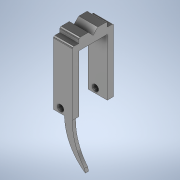
# Autodesk Inventor part: Part2
Saved by Autodesk Inventor 2021 (Build 250183000, 183)
## iProperties
Created: 2020-11-21
Part Number: Part2
Material: Nickel-Copper Alloy 400
Document SubType Name: Modeling
Designer: pedro
Density: 8.83 g/cm^3
Appearance: Cromado - Preto polido
Author: pedro
Autodesk Inventor part; units mm, degrees
ref_plane "YZ Plane" through (0, 0, 0) normal (1, 0, 0) x (0, 1, 0)
ref_plane "XZ Plane" through (0, 0, 0) normal (0, 1, 0) x (-1, 0, 0)
ref_plane "XY Plane" through (0, 0, 0) normal (0, 0, 1) x (1, 0, 0)
sketch "Sketch1" plane through (0, 0, 0) normal (0, 0, 1) x (1, 0, 0)
  line L0 (0, 0) -> (-5, 0)
  line L1 (-5, 0) -> (-5, 20)
  line L2 (-5, 20) -> (0, 20)
  line L3 (0, 20) -> (0, 0)
  arc A0 (0, 0) -> (3.7628, -11.2711) centre (16.9897, -0.5917) ccw
  arc A1 (-2.5, 0) -> (3.7698, -12.1977) centre (12.5, 0) ccw
  line L4 (4.0643, -12.4032) -> (3.7628, -11.2711)
  line L5 (-5, 0) -> (-2.5, 0)
  line L6 (0, 20) -> (0, 0)
  line L7 (3.7698, -12.1977) -> (4.0643, -12.4032)
  circle A2 centre (-3.75, 1.4711) radius 1.0155
  dimension "d0" = 5
  dimension "d1" = 20
  dimension "d2" = 17
  dimension "d3" = 15
  constraints: 16 end point, 5 point on circle, 3 centre point, 2 parallel, 2 perpendicular, 1 collinear, 1 horizontal, 1 midpoint
  measures "d0" distance of L1.end L2.end
  measures "d1" distance of L2.end L0.start
  measures "d2" radius of A0
  measures "d3" radius of A1
extrude "Extrusion1" add sketch "Sketch1" against normal blind 13 contours L0 L1 L2 L3 | A2
extrude "Extrusion2" add sketch "Sketch1" against normal blind 1 contours A0 L4 L7 A1 L0
sketch "Sketch2" plane through (0, 0, -13) normal (1, 0, 0) x (0, 0, -1)
  line L0 (-12, 0) -> (0, 0) projected
  line L1 (-11, 14.4434) -> (-11, 18)
  line L2 (-2, 18) -> (-2, 0)
  line L3 (-2, 0) -> (-11, 0)
  line L4 (-13, 20) -> (0, 20) projected
  line L5 (-13, -11.2711) -> (-12, -11.2711) projected
  line L6 (-4.8653, 18) -> (-2, 18)
  line L7 (-13, 0) -> (-13, 20) projected
  line L8 (0, 20) -> (0, 0) projected
  line L9 (-11, 18) -> (-4.8653, 18)
  line L10 (-11, 14.4434) -> (-11, 0)
  line L11 (-13, 0) -> (0, 0) projected
  line L12 (-11, 20) -> (-11, 21.5)
  line L13 (-2, 21.5) -> (-2, 20)
  line L14 (-11, 20) -> (-2, 20)
  line L15 (-13, 20) -> (0, 20) projected
  line L16 (-6.5, 21.5) -> (-6.5, 20) construction
  line L17 (-5, 21.5) -> (-6.5, 20)
  line L18 (-6.5, 20) -> (-8, 21.5)
  line L19 (-2, 21.5) -> (-5, 21.5)
  line L20 (-8, 21.5) -> (-11, 21.5)
  point P0 (-1, 20)
  point P1 (-12, 20)
  point P2 (-12, 20.7344)
  point P3 (-2, 0)
  dimension "d10" = 18
  dimension "d19" = 2
  dimension "d20" = 2
  dimension "d24" = 2
  dimension "d25" = 4.5
  dimension "d26" = 2
  dimension "d27" = 1.5
  dimension "d28" = 1.5
  constraints: 28 end point, 5 perpendicular, 5 point on line, 3 horizontal, 2 vertical, 1 collinear, 1 midpoint
  measures "d10" distance of L2.start L2.end
  measures "d19" distance between parallel lines of L1 L7
  measures "d20" distance between parallel lines of L8 L2
  measures "d24" distance between parallel lines of L13 L8
  measures "d25" distance between parallel lines of L16 L13
  measures "d26" distance between parallel lines of L7 L12
  measures "d27" distance from line of L16 L17.start
  measures "d28" distance from line of L18.end L16
extrude "Extrusion3" add sketch "Sketch2" against normal blind 5 contours L17 L19 L13 L4
extrude "Extrusion4" add sketch "Sketch2" against normal blind 5 contours L12 L20 L18 L4 | L17 L19 L13 L4
extrude "Extrusion5" cut sketch "Sketch2" against normal through all contours L10 L1 L9 L6 L2 L0
extrude "Extrusion6" cut sketch "Sketch1" against normal through all contours A2
fillet "Arredondamento1" radius 0.5 2 edges at (-2.5, 21.5, -11) (-2.5, 21.5, -2)
fillet "Arredondamento2" radius 0.5 2 edges at (-2.5, 20, -13) (-2.5, 20, 0)
sketch "Esboço3" plane through (-5, 0, -11) normal (-1, 0, 0) x (0, 0, 1)
  arc A0 (11, 19.5) -> (10.5, 20) centre (10.5, 19.5) ccw projected
  line L0 (10.5, 20) -> (9, 20) projected
  line L1 (9, 20) -> (9, 21) projected
  arc A1 (9, 21) -> (8.5, 21.5) centre (8.5, 21) ccw projected
  line L2 (8.5, 21.5) -> (6, 21.5) projected
  line L3 (6, 21.5) -> (4.5, 20) projected
  line L4 (4.5, 20) -> (3, 21.5) projected
  line L5 (3, 21.5) -> (0.5, 21.5) projected
  arc A2 (0.5, 21.5) -> (0, 21) centre (0.5, 21) ccw projected
  line L6 (0, 21) -> (0, 20) projected
  line L7 (0, 20) -> (-1.5, 20) projected
  arc A3 (-1.5, 20) -> (-2, 19.5) centre (-1.5, 19.5) ccw projected
  line L8 (-2, 0) -> (-2, 19.5) projected
  line L9 (0, 0) -> (-2, 0) projected
  line L10 (0, 0) -> (0, 18) projected
  line L11 (0, 18) -> (9, 18) projected
  line L12 (9, 18) -> (9, 0) projected
  line L13 (11, 0) -> (9, 0) projected
  line L14 (11, 19.5) -> (11, 0) projected
  point P0 (11, 0)
extrude "Extrusão7" add sketch "Esboço3" along normal blind 1
body "Solid1"
